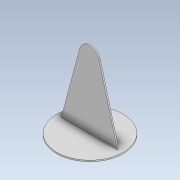
# Autodesk Inventor part: 大yaw
Saved by Autodesk Inventor 2022.5 (Build 265521000, 521)
## iProperties
Created: 2024-11-12
Part Number: 大yaw
Material: 常规
Document SubType Name: Modeling
Designer: Gagouking
Density: 1 g/cm^3
Appearance: 默认
Author: Gagouking
Autodesk Inventor part; units mm, degrees
ref_plane "YZ Plane" through (0, 0, 0) normal (1, 0, 0) x (0, 1, 0)
ref_plane "XZ Plane" through (0, 0, 0) normal (0, 1, 0) x (-1, 0, 0)
ref_plane "XY Plane" through (0, 0, 0) normal (0, 0, 1) x (1, 0, 0)
sketch "草图1" plane through (0, 0, 0) normal (0, 1, 0) x (-1, 0, 0)
  circle A0 centre (0, 0) radius 25
  dimension "d0" = 50
  constraints: 1 centre point, 1 coincident
  measures "d0" diameter of A0
sketch "草图2" plane through (0, 0, 0) normal (0, 0, 1) x (1, 0, 0)
  line L0 (0, 0) -> (0, 50)
  circle A0 centre (0, 50) radius 7.5
  line L1 (-7.2444, 51.9411) -> (-21.43, -1)
  line L2 (-21.43, -1) -> (21.43, -1)
  line L3 (21.43, -1) -> (7.2444, 51.9411)
  line L4 (10, -1) -> (-10, -1)
  dimension "d1" = 50
  dimension "d2" = 15
  dimension "d7" = 30
  constraints: 10 end point, 2 horizontal, 2 point on circle, 2 tangent, 1 centre point, 1 coincident, 1 collinear, 1 vertical, 3 other
  measures "d1" distance of L0.start L0.end
  measures "d2" diameter of A0
  measures "d7" angle of L3 L1
extrude "拉伸1" add sketch "草图1" against normal blind 1
extrude "拉伸2" add sketch "草图2" along normal mid plane 1
